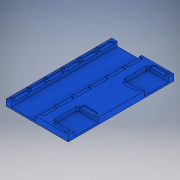
# Autodesk Inventor part: Assembly Plate
Saved by Autodesk Inventor 2019.4 (Build 234330000, 330)
## iProperties
Created: 2021-01-11
Part Number: Assembly Plate
Material: Aluminum, Anodized Blue
Document SubType Name: Modeling
Designer: caleb
Density: 2.7 g/cm^3
Appearance: Anodized - Blue
Author: caleb
Autodesk Inventor part; units mm, degrees
ref_plane "YZ Plane" through (0, 0, 0) normal (1, 0, 0) x (0, 1, 0)
ref_plane "XZ Plane" through (0, 0, 0) normal (0, 1, 0) x (-1, 0, 0)
ref_plane "XY Plane" through (0, 0, 0) normal (0, 0, 1) x (1, 0, 0)
sketch "Sketch1" plane through (0, 0, 0) normal (0, 1, 0) x (-1, 0, 0)
  line L0 (-63.5, 107.95) -> (63.5, 107.95)
  line L1 (63.5, 107.95) -> (63.5, -107.95)
  line L2 (63.5, -107.95) -> (-63.5, -107.95)
  line L3 (-63.5, -107.95) -> (-63.5, 107.95)
  line L4 (-63.5, 107.95) -> (63.5, -107.95) construction
  line L5 (63.5, 107.95) -> (-63.5, -107.95) construction
  point P0 (0, 0)
  dimension "d0" = 127
  dimension "d1" = 215.9
  constraints: 12 end point, 2 midpoint, 2 parallel, 1 horizontal, 1 perpendicular
  measures "d0" distance of L1.end L2.end
  measures "d1" distance of L0.end L1.end
extrude "Extrusion1" add sketch "Sketch1" along normal blind 12.7
sketch "Sketch8" plane through (0, 12.7, 0) normal (0, 1, 0) x (1, 0, 0)
  line L0 (-63.5, -107.95) -> (63.5, -107.95) projected
  line L1 (63.5, 107.95) -> (-63.5, 107.95) projected
  line L2 (-63.5, 107.95) -> (-63.5, -107.95) projected
  line L3 (63.5, -107.95) -> (63.5, 107.95) projected
  line L4 (-52.5, -107.95) -> (-2.5, -107.95)
  line L5 (-2.5, -107.95) -> (-2.5, 107.95)
  line L6 (-2.5, 107.95) -> (-52.5, 107.95)
  line L7 (-52.5, 107.95) -> (-52.5, -107.95)
  point P0 (0, 0)
  dimension "d91" = 11
  dimension "d92" = 50
  constraints: 8 end point, 2 parallel, 2 point on line, 1 horizontal, 1 perpendicular
  measures "d91" distance between parallel lines of L2 L7
  measures "d92" distance between parallel lines of L7 L5
extrude "Extrusion7" cut sketch "Sketch8" against normal blind 9 contours L7 L1 L5 L0
sketch "Sketch9" plane through (0, 12.7, 0) normal (0, 1, 0) x (1, 0, 0)
  line L0 (-63.5, -107.95) -> (-52.5, -107.95) projected
  line L1 (-63.5, 107.95) -> (-63.5, -107.95) projected
  line L2 (-52.5, -107.95) -> (-52.5, 107.95) projected
  line L3 (-52.5, -100.922) -> (-59, -100.922)
  line L4 (-59, -100.922) -> (-59, -74.097)
  line L5 (-55.825, -70.922) -> (-52.5, -70.922)
  line L6 (-52.5, -70.922) -> (-52.5, -100.922)
  circle A0 centre (-59, -100.922) radius 3.175
  line L7 (-2.5, 107.95) -> (-2.5, -107.95) projected
  line L8 (-2.5, -107.95) -> (63.5, -107.95) projected
  line L9 (-2.5, -100.922) -> (2.325, -100.922)
  line L10 (5.5, -97.747) -> (5.5, -74.097)
  line L11 (2.325, -70.922) -> (-2.5, -70.922)
  line L12 (-2.5, -70.922) -> (-2.5, -100.922)
  arc A1 (-55.825, -70.922) -> (-59, -74.097) centre (-55.825, -74.097) ccw
  arc A2 (5.5, -74.097) -> (2.325, -70.922) centre (2.325, -74.097) ccw
  arc A3 (2.325, -100.922) -> (5.5, -97.747) centre (2.325, -97.747) ccw
  arc A4 (5.5, -39.269) -> (2.325, -36.094) centre (2.325, -39.269) ccw
  line L13 (-2.5, -36.094) -> (-2.5, -66.094)
  line L14 (5.5, -62.919) -> (5.5, -39.269)
  line L15 (-2.5, -66.094) -> (2.325, -66.094)
  arc A5 (2.325, -66.094) -> (5.5, -62.919) centre (2.325, -62.919) ccw
  line L16 (2.325, -36.094) -> (-2.5, -36.094)
  line L17 (-52.5, -36.094) -> (-52.5, -66.094)
  line L18 (-55.825, -36.094) -> (-52.5, -36.094)
  arc A6 (-55.825, -36.094) -> (-59, -39.269) centre (-55.825, -39.269) ccw
  line L19 (-59, -66.094) -> (-59, -39.269)
  line L20 (-52.5, -66.094) -> (-59, -66.094)
  circle A7 centre (-59, -66.094) radius 3.175
  arc A8 (5.5, -4.441) -> (2.325, -1.266) centre (2.325, -4.441) ccw
  line L21 (-2.5, -1.266) -> (-2.5, -31.266)
  line L22 (5.5, -28.091) -> (5.5, -4.441)
  line L23 (-2.5, -31.266) -> (2.325, -31.266)
  arc A9 (2.325, -31.266) -> (5.5, -28.091) centre (2.325, -28.091) ccw
  line L24 (2.325, -1.266) -> (-2.5, -1.266)
  line L25 (-52.5, -1.266) -> (-52.5, -31.266)
  line L26 (-55.825, -1.266) -> (-52.5, -1.266)
  arc A10 (-55.825, -1.266) -> (-59, -4.441) centre (-55.825, -4.441) ccw
  line L27 (-59, -31.266) -> (-59, -4.441)
  line L28 (-52.5, -31.266) -> (-59, -31.266)
  circle A11 centre (-59, -31.266) radius 3.175
  arc A12 (5.5, 30.387) -> (2.325, 33.562) centre (2.325, 30.387) ccw
  line L29 (-2.5, 33.562) -> (-2.5, 3.562)
  line L30 (5.5, 6.737) -> (5.5, 30.387)
  line L31 (-2.5, 3.562) -> (2.325, 3.562)
  arc A13 (2.325, 3.562) -> (5.5, 6.737) centre (2.325, 6.737) ccw
  line L32 (2.325, 33.562) -> (-2.5, 33.562)
  line L33 (-52.5, 33.562) -> (-52.5, 3.562)
  line L34 (-55.825, 33.562) -> (-52.5, 33.562)
  arc A14 (-55.825, 33.562) -> (-59, 30.387) centre (-55.825, 30.387) ccw
  line L35 (-59, 3.562) -> (-59, 30.387)
  line L36 (-52.5, 3.562) -> (-59, 3.562)
  circle A15 centre (-59, 3.562) radius 3.175
  arc A16 (5.5, 65.215) -> (2.325, 68.39) centre (2.325, 65.215) ccw
  line L37 (-2.5, 68.39) -> (-2.5, 38.39)
  line L38 (5.5, 41.565) -> (5.5, 65.215)
  line L39 (-2.5, 38.39) -> (2.325, 38.39)
  arc A17 (2.325, 38.39) -> (5.5, 41.565) centre (2.325, 41.565) ccw
  line L40 (2.325, 68.39) -> (-2.5, 68.39)
  line L41 (-52.5, 68.39) -> (-52.5, 38.39)
  line L42 (-55.825, 68.39) -> (-52.5, 68.39)
  arc A18 (-55.825, 68.39) -> (-59, 65.215) centre (-55.825, 65.215) ccw
  line L43 (-59, 38.39) -> (-59, 65.215)
  line L44 (-52.5, 38.39) -> (-59, 38.39)
  circle A19 centre (-59, 38.39) radius 3.175
  arc A20 (5.5, 100.043) -> (2.325, 103.218) centre (2.325, 100.043) ccw
  line L45 (-2.5, 103.218) -> (-2.5, 73.218)
  line L46 (5.5, 76.393) -> (5.5, 100.043)
  line L47 (-2.5, 73.218) -> (2.325, 73.218)
  arc A21 (2.325, 73.218) -> (5.5, 76.393) centre (2.325, 76.393) ccw
  line L48 (2.325, 103.218) -> (-2.5, 103.218)
  line L49 (-52.5, 103.218) -> (-52.5, 73.218)
  line L50 (-55.825, 103.218) -> (-52.5, 103.218)
  arc A22 (-55.825, 103.218) -> (-59, 100.043) centre (-55.825, 100.043) ccw
  line L51 (-59, 73.218) -> (-59, 100.043)
  line L52 (-52.5, 73.218) -> (-59, 73.218)
  circle A23 centre (-59, 73.218) radius 3.175
  point P0 (0, 0)
  point P1 (-59, -70.922)
  point P2 (5.5, -70.922)
  point P3 (5.5, -100.922)
  point P4 (5.5, -36.094)
  point P5 (5.5, -66.094)
  point P6 (-59, -36.094)
  point P7 (5.5, -1.266)
  point P8 (5.5, -31.266)
  point P9 (-59, -1.266)
  point P10 (5.5, 33.562)
  point P11 (5.5, 3.562)
  point P12 (-59, 33.562)
  point P13 (5.5, 68.39)
  point P14 (5.5, 38.39)
  point P15 (-59, 68.39)
  point P16 (5.5, 103.218)
  point P17 (5.5, 73.218)
  point P18 (-59, 103.218)
  dimension "d95" = 7.028
  dimension "d96" = 30
  dimension "d97" = 6.35
  dimension "d99" = 6.5
  dimension "d100" = 7.028
  dimension "d101" = 30
  dimension "d102" = 8
  dimension "d105" = 3.175
  dimension "d108" = 34.828
  constraints: 96 end point, 38 point on line, 36 point on circle, 24 centre point, 6 coincident, 6 tangent, 4 parallel, 2 equal radius, 2 horizontal, 2 perpendicular, 1 vertical, 150 other
  measures "d95" distance between parallel lines of L0 L3
  measures "d96" distance of L3.end point (-59, -70.922)
  measures "d97" diameter of A0
  measures "d99" distance of L3.start L3.end
  measures "d100" distance between parallel lines of L8 L9
  measures "d101" distance of point (5.5, -100.922) point (5.5, -70.922)
  measures "d102" distance of point (5.5, -70.922) L11.end
  measures "d105" radius of A1
  measures "d108" distance of L11.end L13.start
extrude "Extrusion8" cut sketch "Sketch9" against normal blind 2
sketch "Sketch10" plane through (0, 12.7, 0) normal (0, 1, 0) x (1, 0, 0)
  line L0 (63.5, 107.95) -> (63.5, -107.95) projected
  line L1 (63.5, -96.95) -> (24.675, -96.95)
  line L2 (21.5, -93.775) -> (21.5, -50.125)
  line L3 (24.675, -46.95) -> (63.5, -46.95)
  line L4 (63.5, -46.95) -> (63.5, -96.95)
  line L5 (-2.5, -107.95) -> (63.5, -107.95) projected
  line L6 (56.472, -96.95) -> (26.472, -96.95)
  line L7 (26.472, -96.95) -> (26.472, -100.275)
  line L8 (29.647, -103.45) -> (56.472, -103.45)
  line L9 (56.472, -103.45) -> (56.472, -96.95)
  line L10 (56.472, -46.95) -> (26.472, -46.95)
  line L11 (26.472, -46.95) -> (26.472, -42.125)
  line L12 (29.647, -38.95) -> (53.297, -38.95)
  line L13 (56.472, -42.125) -> (56.472, -46.95)
  circle A0 centre (56.472, -103.45) radius 3.175
  arc A1 (26.472, -100.275) -> (29.647, -103.45) centre (29.647, -100.275) ccw
  arc A2 (29.647, -38.95) -> (26.472, -42.125) centre (29.647, -42.125) ccw
  arc A3 (56.472, -42.125) -> (53.297, -38.95) centre (53.297, -42.125) ccw
  arc A4 (24.675, -46.95) -> (21.5, -50.125) centre (24.675, -50.125) ccw
  arc A5 (21.5, -93.775) -> (24.675, -96.95) centre (24.675, -93.775) ccw
  line L14 (63.5, 0) -> (16.2003, 0)
  line L15 (63.5, -107.95) -> (63.5, 107.95)
  line L16 (63.5, 96.95) -> (24.675, 96.95)
  line L17 (21.5, 93.775) -> (21.5, 50.125)
  line L18 (24.675, 46.95) -> (63.5, 46.95)
  line L19 (63.5, 46.95) -> (63.5, 96.95)
  line L20 (56.472, 96.95) -> (26.472, 96.95)
  line L21 (26.472, 96.95) -> (26.472, 100.275)
  line L22 (29.647, 103.45) -> (56.472, 103.45)
  line L23 (56.472, 103.45) -> (56.472, 96.95)
  line L24 (56.472, 46.95) -> (26.472, 46.95)
  line L25 (26.472, 46.95) -> (26.472, 42.125)
  line L26 (29.647, 38.95) -> (53.297, 38.95)
  line L27 (56.472, 42.125) -> (56.472, 46.95)
  circle A6 centre (56.472, 103.45) radius 3.175
  arc A7 (29.647, 103.45) -> (26.472, 100.275) centre (29.647, 100.275) ccw
  arc A8 (26.472, 42.125) -> (29.647, 38.95) centre (29.647, 42.125) ccw
  arc A9 (53.297, 38.95) -> (56.472, 42.125) centre (53.297, 42.125) ccw
  arc A10 (21.5, 50.125) -> (24.675, 46.95) centre (24.675, 50.125) ccw
  arc A11 (24.675, 96.95) -> (21.5, 93.775) centre (24.675, 93.775) ccw
  point P0 (0, 0)
  point P1 (21.5, -46.95)
  point P2 (21.5, -96.95)
  point P3 (26.472, -103.45)
  point P4 (26.472, -38.95)
  point P5 (56.472, -38.95)
  point P6 (21.5, 46.95)
  point P7 (21.5, 96.95)
  point P8 (26.472, 103.45)
  point P9 (26.472, 38.95)
  point P10 (56.472, 38.95)
  dimension "d115" = 50
  dimension "d116" = 11
  dimension "d117" = 42
  dimension "d118" = 7.028
  dimension "d119" = 30
  dimension "d120" = 6.5
  dimension "d121" = 8
  dimension "d122" = 7.028
  dimension "d123" = 30
  dimension "d124" = 6.35
  dimension "d125" = 3.175
  constraints: 52 end point, 30 symmetric about line, 26 point on line, 20 point on circle, 12 centre point, 10 tangent, 6 parallel, 4 equal radius, 4 horizontal, 3 perpendicular, 2 coincident, 1 midpoint, 6 other
  measures "d115" distance of point (21.5, -96.95) point (21.5, -46.95)
  measures "d116" distance between parallel lines of L5 L1
  measures "d117" distance of L1.start point (21.5, -96.95)
  measures "d118" distance between parallel lines of L0 L9
  measures "d119" distance of point (26.472, -103.45) L8.end
  measures "d120" distance between parallel lines of L8 L6
  measures "d121" distance of L10.end point (26.472, -38.95)
  measures "d122" distance between parallel lines of L0 L13
  measures "d123" distance of point (26.472, -38.95) point (56.472, -38.95)
  measures "d124" diameter of A0
  measures "d125" radius of A1
extrude "Extrusion9" cut sketch "Sketch10" against normal blind 9 contours L0 L18 A10 L17 A11 L16 | L0 L1 A5 L2 A4 L3
extrude "Extrusion10" cut sketch "Sketch10" against normal blind 2 contours L16 L21 A7 L22 A6 L23 | L27 A9 L26 A8 L25 L18 | A6 L22 L23 | L23 L22 A6 | L3 L11 A2 L12 A3 L13 | L9 A0 L8 A1 L7 L1 | A0 L8 L9 | L9 L8 A0
body "Solid1"
